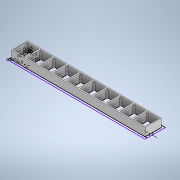
# Autodesk Inventor part: 4x led strip divider
Saved by Autodesk Inventor 2022 (Build 260153000, 153)
## iProperties
Created: 2022-04-12
Part Number: 4x led strip divider
Material: Generic
Document SubType Name: Modeling
Designer: a-dubs
Density: 1 g/cm^3
Appearance: Default
Author: a-dubs
Autodesk Inventor part; units mm, degrees
ref_plane "YZ Plane" through (0, 0, 0) normal (1, 0, 0) x (0, 1, 0)
ref_plane "XZ Plane" through (0, 0, 0) normal (0, 1, 0) x (-1, 0, 0)
ref_plane "XY Plane" through (0, 0, 0) normal (0, 0, 1) x (1, 0, 0)
sketch "Sketch1" plane through (0, 0, 0) normal (0, 1, 0) x (-1, 0, 0)
  line L0 (0, 0) -> (-9.9, 0)
  line L1 (0, 0) -> (0, -10.3)
  line L2 (0, -10.3) -> (-9.9, -10.3)
  line L3 (-9.9, -10.3) -> (-9.9, 0)
  line L4 (-9.9, -10.3) -> (-9.4, -10.3)
  line L5 (-9.4, -10.3) -> (-9.4, 0)
  line L6 (0, -10.3) -> (-0.5, -10.3)
  line L7 (-0.5, -10.3) -> (-0.5, 0)
  line L8 (-0.5, 0.85) -> (-9.9, 0.85)
  line L9 (-9.9, 0.85) -> (-9.9, 0)
  line L10 (0, 0) -> (0, 0.85)
  line L11 (0, 0.85) -> (-0.5, 0.85)
  line L12 (0, -10.3) -> (0, -11.15)
  line L13 (0, -11.15) -> (-9.9, -11.15)
  line L14 (-9.9, -11.15) -> (-9.9, -10.3)
  line L15 (-9.9, -11.15) -> (-19.8, -11.15)
  line L16 (-19.8, -11.15) -> (-19.8, -10.3)
  line L17 (-19.8, -10.3) -> (-19.8, 0)
  line L18 (-19.3, -10.3) -> (-19.3, 0)
  line L19 (-9.9, -10.3) -> (-19.8, -10.3)
  line L20 (-10.4, -10.3) -> (-10.4, 0)
  line L21 (-9.9, 0) -> (-9.9, -10.3)
  line L22 (-9.9, 0) -> (-9.9, 0.85)
  line L23 (-9.9, 0.85) -> (-10.4, 0.85)
  line L24 (-10.4, 0.85) -> (-19.8, 0.85)
  line L25 (-9.9, 0) -> (-19.8, 0)
  line L26 (-19.8, 0.85) -> (-19.8, 0)
  line L27 (-19.8, -11.15) -> (-29.7, -11.15)
  line L28 (-29.7, -11.15) -> (-29.7, -10.3)
  line L29 (-29.7, -10.3) -> (-29.7, 0)
  line L30 (-29.2, -10.3) -> (-29.2, 0)
  line L31 (-19.8, -10.3) -> (-29.7, -10.3)
  line L32 (-20.3, -10.3) -> (-20.3, 0)
  line L33 (-19.8, 0) -> (-19.8, -10.3)
  line L34 (-19.8, 0) -> (-19.8, 0.85)
  line L35 (-19.8, 0.85) -> (-20.3, 0.85)
  line L36 (-20.3, 0.85) -> (-29.7, 0.85)
  line L37 (-19.8, 0) -> (-29.7, 0)
  line L38 (-29.7, 0.85) -> (-29.7, 0)
  line L39 (-29.7, -11.15) -> (-39.6, -11.15)
  line L40 (-39.6, -11.15) -> (-39.6, -10.3)
  line L41 (-39.6, -10.3) -> (-39.6, 0)
  line L42 (-39.1, -10.3) -> (-39.1, 0)
  line L43 (-29.7, -10.3) -> (-39.6, -10.3)
  line L44 (-30.2, -10.3) -> (-30.2, 0)
  line L45 (-29.7, 0) -> (-29.7, -10.3)
  line L46 (-29.7, 0) -> (-29.7, 0.85)
  line L47 (-29.7, 0.85) -> (-30.2, 0.85)
  line L48 (-30.2, 0.85) -> (-39.6, 0.85)
  line L49 (-29.7, 0) -> (-39.6, 0)
  line L50 (-39.6, 0.85) -> (-39.6, 0)
  line L51 (-39.6, -11.15) -> (-49.5, -11.15)
  line L52 (-49.5, -11.15) -> (-49.5, -10.3)
  line L53 (-49.5, -10.3) -> (-49.5, 0)
  line L54 (-49, -10.3) -> (-49, 0)
  line L55 (-39.6, -10.3) -> (-49.5, -10.3)
  line L56 (-40.1, -10.3) -> (-40.1, 0)
  line L57 (-39.6, 0) -> (-39.6, -10.3)
  line L58 (-39.6, 0) -> (-39.6, 0.85)
  line L59 (-39.6, 0.85) -> (-40.1, 0.85)
  line L60 (-40.1, 0.85) -> (-49.5, 0.85)
  line L61 (-39.6, 0) -> (-49.5, 0)
  line L62 (-49.5, 0.85) -> (-49.5, 0)
  line L63 (-49.5, -11.15) -> (-59.4, -11.15)
  line L64 (-59.4, -11.15) -> (-59.4, -10.3)
  line L65 (-59.4, -10.3) -> (-59.4, 0)
  line L66 (-58.9, -10.3) -> (-58.9, 0)
  line L67 (-49.5, -10.3) -> (-59.4, -10.3)
  line L68 (-50, -10.3) -> (-50, 0)
  line L69 (-49.5, 0) -> (-49.5, -10.3)
  line L70 (-49.5, 0) -> (-49.5, 0.85)
  line L71 (-49.5, 0.85) -> (-50, 0.85)
  line L72 (-50, 0.85) -> (-59.4, 0.85)
  line L73 (-49.5, 0) -> (-59.4, 0)
  line L74 (-59.4, 0.85) -> (-59.4, 0)
  line L75 (-59.4, -11.15) -> (-69.3, -11.15)
  line L76 (-69.3, -11.15) -> (-69.3, -10.3)
  line L77 (-69.3, -10.3) -> (-69.3, 0)
  line L78 (-68.8, -10.3) -> (-68.8, 0)
  line L79 (-59.4, -10.3) -> (-69.3, -10.3)
  line L80 (-59.9, -10.3) -> (-59.9, 0)
  line L81 (-59.4, 0) -> (-59.4, -10.3)
  line L82 (-59.4, 0) -> (-59.4, 0.85)
  line L83 (-59.4, 0.85) -> (-59.9, 0.85)
  line L84 (-59.9, 0.85) -> (-69.3, 0.85)
  line L85 (-59.4, 0) -> (-69.3, 0)
  line L86 (-69.3, 0.85) -> (-69.3, 0)
  line L87 (-69.3, -11.15) -> (-79.2, -11.15)
  line L88 (-79.2, -11.15) -> (-79.2, -10.3)
  line L89 (-79.2, -10.3) -> (-79.2, 0)
  line L90 (-78.7, -10.3) -> (-78.7, 0)
  line L91 (-69.3, -10.3) -> (-79.2, -10.3)
  line L92 (-69.8, -10.3) -> (-69.8, 0)
  line L93 (-69.3, 0) -> (-69.3, -10.3)
  line L94 (-69.3, 0) -> (-69.3, 0.85)
  line L95 (-69.3, 0.85) -> (-69.8, 0.85)
  line L96 (-69.8, 0.85) -> (-79.2, 0.85)
  line L97 (-69.3, 0) -> (-79.2, 0)
  line L98 (-79.2, 0.85) -> (-79.2, 0)
  line L99 (-79.2, -11.15) -> (-89.1, -11.15)
  line L100 (-89.1, -11.15) -> (-89.1, -10.3)
  line L101 (-89.1, -10.3) -> (-89.1, 0)
  line L102 (-88.6, -10.3) -> (-88.6, 0)
  line L103 (-79.2, -10.3) -> (-89.1, -10.3)
  line L104 (-79.7, -10.3) -> (-79.7, 0)
  line L105 (-79.2, 0) -> (-79.2, -10.3)
  line L106 (-79.2, 0) -> (-79.2, 0.85)
  line L107 (-79.2, 0.85) -> (-79.7, 0.85)
  line L108 (-79.7, 0.85) -> (-89.1, 0.85)
  line L109 (-79.2, 0) -> (-89.1, 0)
  line L110 (-89.1, 0.85) -> (-89.1, 0)
  line L111 (-89.1, -11.15) -> (-99, -11.15)
  line L112 (-99, -11.15) -> (-99, -10.3)
  line L113 (-99, -10.3) -> (-99, 0)
  line L114 (-98.5, -10.3) -> (-98.5, 0)
  line L115 (-89.1, -10.3) -> (-99, -10.3)
  line L116 (-89.6, -10.3) -> (-89.6, 0)
  line L117 (-89.1, 0) -> (-89.1, -10.3)
  line L118 (-89.1, 0) -> (-89.1, 0.85)
  line L119 (-89.1, 0.85) -> (-89.6, 0.85)
  line L120 (-89.6, 0.85) -> (-99, 0.85)
  line L121 (-89.1, 0) -> (-99, 0)
  line L122 (-99, 0.85) -> (-99, 0)
  line L123 (0, -11.15) -> (0, 0.85)
  line L124 (0, -11.15) -> (0, -12.65)
  line L125 (0, -12.65) -> (1.5, -12.65)
  line L126 (-99, 0.85) -> (-100.5, 0.85)
  line L127 (-100.5, 0.85) -> (-100.5, 2.35)
  line L128 (1.5, -12.65) -> (-100.5, -12.65)
  line L129 (-100.5, -12.65) -> (-100.5, 2.35)
  line L130 (-100.5, 2.35) -> (1.5, 2.35)
  line L131 (1.5, 2.35) -> (1.5, -12.65)
  line L132 (0, -11.15) -> (1.5, -11.15)
  line L133 (0, 0.85) -> (1.5, 0.85)
  line L134 (0, -11.15) -> (-2, -11.15)
  line L135 (-2, -11.15) -> (-2, 0.85)
  line L136 (-0.5, -10.3) -> (-1.5, -10.3)
  line L137 (-1.5, -10.3) -> (-0.5, -9.3)
  line L138 (-9.4, -10.3) -> (-8.4, -10.3)
  line L139 (-8.4, -10.3) -> (-9.4, -9.3)
  line L140 (-9.4, 0) -> (-9.4, -1)
  line L141 (-9.4, -1) -> (-8.4, 0)
  line L142 (-2, 0) -> (-3, 0)
  line L143 (-0.5, 0) -> (-1.5, 0)
  line L144 (-1.5, 0) -> (-0.5, -1)
  dimension "d0" = 9.9
  dimension "d1" = 10.3
  dimension "d2" = 0.5
  dimension "d3" = 0.5
  dimension "d6" = 0.85
  dimension "d7" = 0.85
  dimension "d10" = 9.9
  dimension "d15" = 1.5
  dimension "d16" = 1.5
  dimension "d19" = 1.5
  dimension "d20" = 2
  dimension "d26" = 1
  dimension "d27" = 45
  dimension "d28" = 1
  dimension "d29" = 1
  dimension "d30" = 1
  dimension "d31" = 1
  constraints: 290 end point, 65 point on line, 14 perpendicular, 4 horizontal, 3 parallel, 2 collinear, 2 vertical, 224 other
  measures "d0" distance of L0.start L0.end
  measures "d1" distance of L0.start L1.end
  measures "d2" distance of L2.end L4.end
  measures "d3" distance of L1.end L6.end
  measures "d6" distance of L0.start L10.end
  measures "d7" distance of L1.end L12.end
  measures "d10" distance of L12.end L15.start
  measures "d15" distance of L12.end L124.end
  measures "d16" distance of L124.end L125.end
  measures "d19" distance of L120.end L126.end
  measures "d20" distance of L12.end L134.end
  measures "d26" distance of L6.end L136.end
  measures "d27" angle of L136 L137
  measures "d28" distance of L4.end L138.end
  measures "d29" distance of L5.end L140.end
  measures "d30" distance of L142.start L142.end
  measures "d31" distance of L7.end L143.end
extrude "Extrusion1" add sketch "Sketch1" along normal blind 6 contours L1 L2 L7 L0 | L0 L135 L8 L11 L10 | L12 L13 L135 L2 | L0 L9 L8 L135 | L13 L14 L2 L135 | L3 L0 L5 L2
extrude "Extrusion2" add sketch "Sketch1" along normal blind 5 contours L7 L144 L0 | L2 L137 L7 | L141 L5 L0 | L2 L5 L139
pattern_linear "Rectangular Pattern1" count 10 spacing 9.9 along (1, 0, 0) of "Extrusion1", "Extrusion2"
equation "\"d25\" = d10"
body "Solid1"
